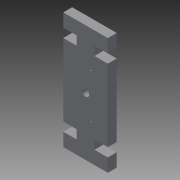
# Autodesk Inventor part: predni_komatex(0)
Saved by Autodesk Inventor 2015 (Build 190159000, 159)
## iProperties
Created: 2015-01-01
Part Number: predni_komatex(0)
Material: Generic
Document SubType Name: Modeling
Designer: Turboslimak
Density: 1 g/cm^3
Appearance: Default
Author: Turboslimak
Autodesk Inventor part; units mm, degrees
ref_plane "YZ Plane" through (0, 0, 0) normal (1, 0, 0) x (0, 1, 0)
ref_plane "XZ Plane" through (0, 0, 0) normal (0, 1, 0) x (-1, 0, 0)
ref_plane "XY Plane" through (0, 0, 0) normal (0, 0, 1) x (1, 0, 0)
sketch "Sketch1" plane through (0, 0, 0) normal (0, 1, 0) x (-1, 0, 0)
  line L0 (25, -65.5) -> (-25, -65.5)
  line L1 (-25, 65.5) -> (25, 65.5)
  circle A0 centre (0, 0) radius 4
  circle A1 centre (-6, -25) radius 1
  circle A2 centre (-6, 25) radius 1
  line L2 (-25, 65.5) -> (-10, 65.5)
  line L3 (-10, 50.6) -> (-25, 50.6)
  line L4 (-25, 50.6) -> (-25, 65.5)
  line L5 (-25, 65.5) -> (-10, 65.5)
  line L6 (-10, 40.6) -> (-25, 40.6)
  line L7 (-25, -65.5) -> (-10, -65.5)
  line L8 (-10, -40.6) -> (-25, -40.6)
  line L9 (-25, -65.5) -> (-10, -65.5)
  line L10 (-10, -50.6) -> (-25, -50.6)
  line L11 (-25, -50.6) -> (-25, -65.5)
  line L12 (25, -65.5) -> (10, -65.5)
  line L13 (10, -40.6) -> (25, -40.6)
  line L14 (25, -65.5) -> (10, -65.5)
  line L15 (10, -50.6) -> (25, -50.6)
  line L16 (25, -50.6) -> (25, -65.5)
  line L17 (25, 65.5) -> (10, 65.5)
  line L18 (10, 40.6) -> (25, 40.6)
  line L19 (25, 65.5) -> (10, 65.5)
  line L20 (10, 50.6) -> (25, 50.6)
  line L21 (25, 50.6) -> (25, 65.5)
  line L22 (-10, 50.6) -> (-10, 40.6)
  line L23 (-25, 40.6) -> (-25, -40.6)
  line L24 (-10, -40.6) -> (-10, -50.6)
  line L25 (10, -40.6) -> (10, -50.6)
  line L26 (25, -40.6) -> (25, 40.6)
  line L27 (10, 40.6) -> (10, 50.6)
  dimension "d0" = 50
  dimension "d1" = 131
  dimension "d4" = 8
  dimension "d10" = 2
  dimension "d18" = 14.9
  dimension "d19" = 15
  dimension "d20" = 24.9
  dimension "d21" = 15
  dimension "d22" = 24.9
  dimension "d24" = 14.9
  dimension "d25" = 15
  dimension "d26" = 24.9
  dimension "d28" = 14.9
  dimension "d29" = 15
  dimension "d30" = 24.9
  dimension "d32" = 14.9
  constraints: 56 end point, 13 parallel, 9 horizontal, 3 centre point, 2 vertical, 1 coincident
  measures "d0" distance of L1.start L1.end
  measures "d1" distance of L0.end L1.start
  measures "d4" diameter of A0
  measures "d10" diameter of A2
  measures "d18" distance of L2.end L3.start
  measures "d19" distance of L6.start L6.end
  measures "d20" distance of L5.end L6.start
  measures "d21" distance of L8.end L8.start
  measures "d22" distance of L8.start L7.end
  measures "d24" distance of L10.start L9.end
  measures "d25" distance of L13.start L13.end
  measures "d26" distance of L12.end L13.start
  measures "d28" distance of L14.end L15.start
  measures "d29" distance of L18.end L18.start
  measures "d30" distance of L18.start L17.end
  measures "d32" distance of L20.start L19.end
extrude "Extrusion1" add sketch "Sketch1" along normal blind 10 contours L0 L11 L10 L24 L8 L23 L6 L22 L3 L4 L1 L21 L20 L27 L18 L26 L13 L25 L15 L16 | A0 | A1 | A2
extrude "Extrusion2" cut sketch "Sketch1" along normal blind 10 contours A0 | A1 | A2
sketch "Sketch3" plane through (-25, 0, -40.6) normal (-1, 0, 0) x (0, 0, 1)
  circle A0 centre (40.6, 5) radius 1.25
  point P0 (40.6, 0)
  dimension "d34" = 2.5
  constraints: 1 centre point
  measures "d34" diameter of A0
extrude "Extrusion4" cut sketch "Sketch3" against normal blind 10
body "Solid1"
